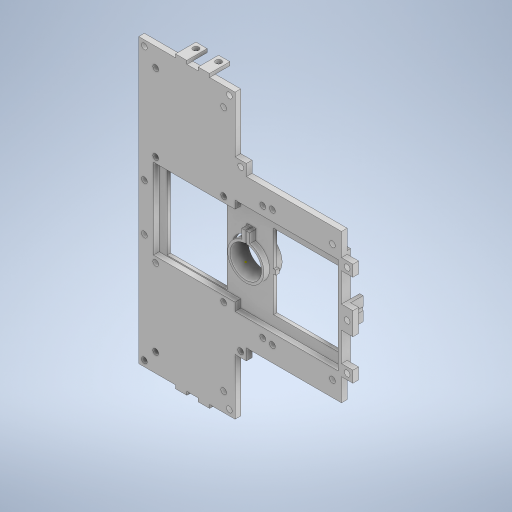
# Autodesk Inventor part: RoverMainHousing
Saved by Autodesk Inventor 2024 (Build 280153000, 153)
## iProperties
Created: 2025-11-13
Part Number: RoverMainHousing
Material: Generic
Document SubType Name: Modeling
Designer: albah
Density: 1 g/cm^3
Appearance: Default
Author: albah
Autodesk Inventor part; units mm, degrees
ref_plane "YZ Plane" through (0, 0, 0) normal (1, 0, 0) x (0, 1, 0)
ref_plane "XZ Plane" through (0, 0, 0) normal (0, 1, 0) x (-1, 0, 0)
ref_plane "XY Plane" through (0, 0, 0) normal (0, 0, 1) x (1, 0, 0)
sketch "Sketch1" plane through (0, 0, 0) normal (0, 0, 1) x (1, 0, 0)
  line L0 (-81.5, 42.5) -> (81.5, 42.5)
  line L1 (81.5, 42.5) -> (81.5, -42.5)
  line L2 (81.5, -42.5) -> (-81.5, -42.5)
  line L3 (-81.5, -42.5) -> (-81.5, 42.5)
  line L4 (-81.5, 42.5) -> (81.5, -42.5) construction
  line L5 (81.5, 42.5) -> (-81.5, -42.5) construction
  line L6 (84.5, 45.5) -> (-84.5, 45.5)
  line L7 (-84.5, 45.5) -> (-84.5, -45.5)
  line L8 (-84.5, -45.5) -> (84.5, -45.5)
  line L9 (84.5, -45.5) -> (84.5, 45.5)
  line L10 (-84.5, 45.5) -> (-84.5, 65.5)
  line L11 (-84.5, 65.5) -> (84.5, 65.5)
  line L12 (84.5, 65.5) -> (84.5, 45.5)
  line L13 (-84.5, -45.5) -> (-84.5, -65.5)
  line L14 (-84.5, -65.5) -> (84.5, -65.5)
  line L15 (84.5, -65.5) -> (84.5, -45.5)
  point P0 (0, 0)
  dimension "d0" = 163
  dimension "d1" = 85
  dimension "d4" = 3
  dimension "d167" = 20
  dimension "d168" = 20
  constraints: 32 end point, 6 perpendicular, 4 parallel, 2 midpoint, 2 point on line, 1 horizontal, 1 vertical, 3 other
  measures "d0" distance of L0.start L0.end
  measures "d1" distance of L0.end L1.end
  measures "d4" distance between parallel lines of L0 L6
  measures "d167" distance of L6.end L10.end
  measures "d168" distance of L7.end L13.end
extrude "Extrusion1" add sketch "Sketch1" along normal blind 3 contours L0 L1 L2 L3
extrude "Extrusion2" add sketch "Sketch1" along normal blind 8 contours L9 L8 L7 L6
sketch "Sketch2" plane through (0, 0, 8) normal (0, 0, 1) x (1, 0, 0)
  point P0 (0, 0)
sketch "Sketch3" plane through (0, 0, 3) normal (0, 0, 1) x (1, 0, 0)
  circle A0 centre (0, 0) radius 13.85
  circle A1 centre (0, 0) radius 16
  line L0 (0, 16) -> (0, 24)
  line L1 (0.5, 24.0267) -> (-0.5, 24.0267)
  line L2 (-0.5, 24.0267) -> (-0.5, 15.9733)
  line L3 (-0.5, 15.9733) -> (0.5, 15.9733)
  line L4 (0.5, 15.9733) -> (0.5, 24.0267)
  line L5 (0.5, 24.0267) -> (-0.5, 15.9733) construction
  line L6 (-0.5, 24.0267) -> (0.5, 15.9733) construction
  line L7 (-0.5, 24.0267) -> (-3.5, 24.0267)
  line L8 (-3.5, 24.0267) -> (-3.5, 15.6125)
  line L9 (0.5, 24.0267) -> (3.5, 24.0267)
  line L10 (3.5, 24.0267) -> (3.5, 15.6125)
  line L11 (0.5, 15.9733) -> (0.5, 13.841)
  line L12 (-0.5, 15.9733) -> (-0.5, 13.841)
  circle A2 centre (0, 0) radius 17.5
  line L13 (0, -17.5) -> (0, -16)
  line L14 (4, 15) -> (4, 25)
  line L15 (4, 25) -> (-4, 25)
  line L16 (-4, 25) -> (-4, 15)
  line L17 (-4, 15) -> (4, 15)
  line L18 (4, 15) -> (-4, 25) construction
  line L19 (4, 25) -> (-4, 15) construction
  point P0 (0, 20)
  point P1 (3.5, 17.1464)
  point P2 (4, 17.0367)
  point P3 (-4, 17.0367)
  point P4 (-3.5, 17.1464)
  point P5 (4, 15.4919)
  dimension "d15" = 35
  dimension "d7" = 27.7
  dimension "d8" = 32
  dimension "d9" = 8
  dimension "d10" = 1
  dimension "d11" = 3
  dimension "d12" = 3
  dimension "d16" = 10
  dimension "d17" = 8
  constraints: 40 end point, 6 perpendicular, 6 point on circle, 5 midpoint, 5 parallel, 3 coincident, 3 vertical, 2 centre point, 1 horizontal, 3 other
  measures "d7" diameter of A0
  measures "d8" diameter of A1
  measures "d9" distance of L0.start L0.end
  measures "d10" distance of L1.start L1.end
  measures "d11" distance of L1.end L7.end
  measures "d12" distance of L1.start L9.end
  measures "d16" distance of L14.start L14.end
  measures "d17" distance of L15.end L14.end
extrude "Extrusion3" cut sketch "Sketch3" against normal blind 8 contours A0 | A0 L12 L17 L11 | L17 L12 L3 L11 | L3 L2 A1 L4 | A1 L0 A2 L4 | L2 A2 L0 A1 | A2 L2 L1 L4 | A2 L10 L9 L1 L7 L8 L16 L15 L14
extrude "Extrusion4" cut sketch "Sketch3" against normal blind 8 contours L16 A2 L8 A1 | A1 L13 A2 L16
extrude "Extrusion5" add sketch "Sketch3" along normal blind 15 contours A0 L11 L17 L14 A1 L16 L12 | L11 L4 A1 L14 L17 | L17 L16 A1 L2 L12 | L4 A2 L10 A1 | A1 L8 A2 L2 | L4 L9 L10 A2 | A2 L8 L7 L2
extrude "Extrusion6" cut sketch "Sketch3" against normal blind 10 contours A1 L10 A2 L14
sketch "Sketch4" plane through (-3.5, 15.6125, 0) normal (-1, 0, 0) x (0, 0, 1)
  circle A0 centre (12, 4.4142) radius 2.5
  line L0 (18, 8.4142) -> (18, 0) projected
  line L1 (18, 8.4142) -> (0, 8.4142) projected
  point P0 (0, -15.6125)
  point P1 (18, 4.2071)
  dimension "d24" = 5
  dimension "d25" = 6
  dimension "d26" = 4
  constraints: 1 centre point, 1 midpoint
  measures "d24" diameter of A0
  measures "d25" horizontal distance of point (18, 4.207) A0.centre
  measures "d26" distance from line of L1 A0.centre
extrude "Extrusion7" cut sketch "Sketch4" against normal blind 10
sketch "Sketch5" plane through (0, 0, 8) normal (0, 0, 1) x (1, 0, 0)
  line L0 (84.5, -45.5) -> (84.5, 45.5) projected
  line L1 (84.5, 45.5) -> (84.5, 35.5)
  line L2 (84.5, 35.5) -> (94.5, 35.5)
  line L3 (94.5, 35.5) -> (94.5, 45.5)
  line L4 (94.5, 45.5) -> (84.5, 45.5)
  line L5 (84.5, -45.5) -> (84.5, -35.5)
  line L6 (84.5, -35.5) -> (94.5, -35.5)
  line L7 (94.5, -35.5) -> (94.5, -45.5)
  line L8 (94.5, -45.5) -> (84.5, -45.5)
  line L9 (-84.5, 45.5) -> (-84.5, -45.5) projected
  line L10 (-84.5, -45.5) -> (-84.5, -35.5)
  line L11 (-84.5, -35.5) -> (-94.5, -35.5)
  line L12 (-94.5, -35.5) -> (-94.5, -45.5)
  line L13 (-94.5, -45.5) -> (-84.5, -45.5)
  line L14 (-84.5, 45.5) -> (-84.5, 35.5)
  line L15 (-84.5, 35.5) -> (-94.5, 35.5)
  line L16 (-94.5, 35.5) -> (-94.5, 45.5)
  line L17 (-94.5, 45.5) -> (-84.5, 45.5)
  line L18 (-84.5, -45.5) -> (84.5, -45.5) projected
  line L19 (84.5, -45.5) -> (74.5, -45.5)
  line L20 (74.5, -45.5) -> (74.5, -55.5)
  line L21 (74.5, -55.5) -> (84.5, -55.5)
  line L22 (84.5, -55.5) -> (84.5, -45.5)
  line L23 (-84.5, -45.5) -> (-84.5, -55.5)
  line L24 (-84.5, -55.5) -> (-74.5, -55.5)
  line L25 (-74.5, -55.5) -> (-74.5, -45.5)
  line L26 (-74.5, -45.5) -> (-84.5, -45.5)
  line L27 (84.5, 45.5) -> (74.5, 45.5)
  line L28 (74.5, 45.5) -> (74.5, 55.5)
  line L29 (74.5, 55.5) -> (84.5, 55.5)
  line L30 (84.5, 55.5) -> (84.5, 45.5)
  line L31 (-84.5, 45.5) -> (-74.5, 45.5)
  line L32 (-74.5, 45.5) -> (-74.5, 55.5)
  line L33 (-74.5, 55.5) -> (-84.5, 55.5)
  line L34 (-84.5, 55.5) -> (-84.5, 45.5)
  line L35 (84.5, 0) -> (84.5, -10)
  line L36 (84.5, -10) -> (94.5, -10)
  line L37 (94.5, -10) -> (94.5, 0)
  line L38 (94.5, 0) -> (84.5, 0)
  line L39 (84.5, 0) -> (84.5, 10)
  line L40 (84.5, 10) -> (94.5, 10)
  line L41 (94.5, 10) -> (94.5, 0)
  line L42 (94.5, 0) -> (84.5, 0)
  line L43 (-74.5, 45.5) -> (-54.5, 45.5)
  line L44 (84.5, 45.5) -> (-84.5, 45.5) projected
  line L45 (-74.5, -45.5) -> (-54.5, -45.5)
  line L46 (-54.5, 45.5) -> (-44.5, 45.5)
  line L47 (-44.5, 45.5) -> (-44.5, 55.5)
  line L48 (-44.5, 55.5) -> (-54.5, 55.5)
  line L49 (-54.5, 55.5) -> (-54.5, 45.5)
  line L50 (-54.5, -45.5) -> (-44.5, -45.5)
  line L51 (-44.5, -45.5) -> (-44.5, -55.5)
  line L52 (-44.5, -55.5) -> (-54.5, -55.5)
  line L53 (-54.5, -55.5) -> (-54.5, -45.5)
  line L54 (74.5, 45.5) -> (54.5, 45.5)
  line L55 (74.5, -45.5) -> (54.5, -45.5)
  line L56 (54.5, -45.5) -> (44.5, -45.5)
  line L57 (44.5, -45.5) -> (44.5, -55.5)
  line L58 (44.5, -55.5) -> (54.5, -55.5)
  line L59 (54.5, -55.5) -> (54.5, -45.5)
  line L60 (54.5, 45.5) -> (44.5, 45.5)
  line L61 (44.5, 45.5) -> (44.5, 55.5)
  line L62 (44.5, 55.5) -> (54.5, 55.5)
  line L63 (54.5, 55.5) -> (54.5, 45.5)
  line L64 (0, -45.5) -> (10, -45.5)
  line L65 (0, -45.5) -> (-10, -45.5)
  line L66 (0, 45.5) -> (10, 45.5)
  line L67 (0, 45.5) -> (-10, 45.5)
  line L68 (10, -45.5) -> (20, -45.5)
  line L69 (20, -45.5) -> (20, -55.5)
  line L70 (20, -55.5) -> (10, -55.5)
  line L71 (10, -55.5) -> (10, -45.5)
  line L72 (-10, -45.5) -> (-20, -45.5)
  line L73 (-20, -45.5) -> (-20, -55.5)
  line L74 (-20, -55.5) -> (-10, -55.5)
  line L75 (-10, -55.5) -> (-10, -45.5)
  line L76 (10, 45.5) -> (20, 45.5)
  line L77 (20, 45.5) -> (20, 55.5)
  line L78 (20, 55.5) -> (10, 55.5)
  line L79 (10, 55.5) -> (10, 45.5)
  line L80 (-10, 45.5) -> (-20, 45.5)
  line L81 (-20, 45.5) -> (-20, 55.5)
  line L82 (-20, 55.5) -> (-10, 55.5)
  line L83 (-10, 55.5) -> (-10, 45.5)
  dimension "d29" = 10
  dimension "d30" = 10
  dimension "d31" = 10
  dimension "d32" = 10
  dimension "d33" = 10
  dimension "d34" = 10
  dimension "d35" = 10
  dimension "d36" = 10
  dimension "d37" = 10
  dimension "d38" = 10
  dimension "d39" = 10
  dimension "d40" = 10
  dimension "d41" = 10
  dimension "d42" = 10
  dimension "d43" = 10
  dimension "d44" = 10
  dimension "d45" = 10
  dimension "d46" = 10
  dimension "d47" = 10
  dimension "d48" = 10
  dimension "d51" = 20
  dimension "d52" = 20
  dimension "d53" = 10
  dimension "d54" = 10
  dimension "d55" = 10
  dimension "d56" = 10
  dimension "d57" = 20
  dimension "d58" = 20
  dimension "d59" = 10
  dimension "d60" = 10
  dimension "d61" = 10
  dimension "d62" = 10
  dimension "d63" = 10
  dimension "d64" = 10
  dimension "d65" = 10
  dimension "d66" = 10
  dimension "d67" = 10
  dimension "d68" = 10
  dimension "d69" = 10
  dimension "d70" = 10
  dimension "d71" = 10
  dimension "d72" = 10
  dimension "d73" = 10
  dimension "d74" = 64.5
  constraints: 160 end point, 36 parallel, 18 perpendicular, 9 point on line, 1 midpoint, 21 other
  measures "d29" distance of L0.end L1.end
  measures "d30" distance of L2.end L1.end
  measures "d31" distance of L0.start L5.end
  measures "d32" distance of L5.end L6.end
  measures "d33" distance of L9.end L10.end
  measures "d34" distance of L11.end L10.end
  measures "d35" distance of L9.start L14.end
  measures "d36" distance of L14.end L15.end
  measures "d37" distance of L0.start L19.end
  measures "d38" distance of L20.end L19.end
  measures "d39" distance of L9.end L23.end
  measures "d40" distance of L24.end L23.end
  measures "d41" distance of L0.end L27.end
  measures "d42" distance of L27.end L28.end
  measures "d43" distance of L9.start L31.end
  measures "d44" distance of L32.end L31.end
  measures "d45" distance of L35.start L35.end
  measures "d46" distance of L36.end L35.end
  measures "d47" distance of L35.start L39.end
  measures "d48" distance of L39.end L40.end
  measures "d51" distance of L31.end L43.end
  measures "d52" distance of L25.end L45.end
  measures "d53" distance of L43.end L46.end
  measures "d54" distance of L47.end L46.end
  measures "d55" distance of L45.end L50.end
  measures "d56" distance of L50.end L51.end
  measures "d57" distance of L27.end L54.end
  measures "d58" distance of L19.end L55.end
  measures "d59" distance of L55.end L56.end
  measures "d60" distance of L57.end L56.end
  measures "d61" distance of L54.end L60.end
  measures "d62" distance of L60.end L61.end
  measures "d63" distance of L64.start L64.end
  measures "d64" distance of L64.start L65.end
  measures "d65" distance of L66.start L67.end
  measures "d66" distance of L64.end L68.end
  measures "d67" distance of L68.end L69.end
  measures "d68" distance of L65.end L72.end
  measures "d69" distance of L73.end L72.end
  measures "d70" distance of L66.end L76.end
  measures "d71" distance of L77.end L76.end
  measures "d72" distance of L67.end L80.end
  measures "d73" distance of L80.end L81.end
  measures "d74" distance between parallel lines of L77 L0
extrude "Extrusion8" add sketch "Sketch5" against normal blind 5 contours L0 L6 L7 L8 | L22 L21 L20 L18 | L0 L38 L37 L36 | L59 L58 L57 L18 | L0 L40 L41 L38 | L69 L70 L71 L18 | L0 L4 L3 L2 | L27 L28 L29 L30 | L75 L74 L73 L18 | L44 L61 L62 L63 | L51 L52 L53 L18 | L44 L79 L78 L77 | L25 L24 L23 L18 | L13 L12 L11 L9 | L44 L81 L82 L83 | L15 L16 L17 L9 | L44 L49 L48 L47 | L34 L33 L32 L31
ref_plane "Work Plane1" through (0, 0, -6) normal (0, 0, -1) x (-1, 0, 0)
sketch "Sketch7" plane through (0, 0, -6) normal (0, 0, -1) x (-1, 0, 0)
  line L0 (-19.5, -35) -> (-19.5, 35)
  line L1 (-19.5, 35) -> (-79.5, 35)
  line L2 (-79.5, 35) -> (-79.5, -35)
  line L3 (-79.5, -35) -> (-19.5, -35)
  line L4 (-19.5, -35) -> (-79.5, 35) construction
  line L5 (-19.5, 35) -> (-79.5, -35) construction
  line L6 (0, 0) -> (-84.5, 0)
  line L7 (-84.5, -45.5) -> (-84.5, 45.5) projected
  line L8 (-79.5, 35) -> (-19.5, 35)
  line L9 (-19.5, 35) -> (-19.5, 33)
  line L10 (-19.5, 33) -> (-79.5, 33)
  line L11 (-79.5, 33) -> (-79.5, 35)
  line L12 (-79.5, -35) -> (-19.5, -35)
  line L13 (-19.5, -35) -> (-19.5, -33)
  line L14 (-19.5, -33) -> (-79.5, -33)
  line L15 (-79.5, -33) -> (-79.5, -35)
  line L16 (-19.5, 0) -> (-19.5, 2)
  line L17 (-19.5, 2) -> (-21.5, 2)
  line L18 (-21.5, 2) -> (-21.5, 0)
  line L19 (-21.5, 0) -> (-19.5, 0)
  line L20 (-21.5, 0) -> (-21.5, -2)
  line L21 (-16.5, 0) -> (-21.5, 0)
  line L22 (-79.5, 0) -> (-79.5, 2)
  line L23 (-79.5, 2) -> (-77.5, 2)
  line L24 (-77.5, 2) -> (-77.5, 0)
  line L25 (-77.5, 0) -> (-79.5, 0)
  line L26 (-79.5, 0) -> (-79.5, -2)
  line L27 (-79.5, -2) -> (-77.5, -2)
  line L28 (-77.5, -2) -> (-77.5, 0)
  line L29 (-77.5, 0) -> (-79.5, 0)
  line L30 (-21.5, -2) -> (-19.5, -2)
  point P0 (-49.5, 0)
  point P1 (-49.5, 0)
  point P2 (-49.5, 0)
  point P3 (-77.5, 0)
  dimension "d78" = 70
  dimension "d79" = 60
  dimension "d80" = 35
  dimension "d81" = 2
  dimension "d82" = 2
  dimension "d83" = 2
  dimension "d84" = 2
  dimension "d85" = 2
  dimension "d87" = 2
  dimension "d88" = 2
  dimension "d89" = 2
  dimension "d90" = 2
  constraints: 60 end point, 14 equal length, 8 point on line, 7 midpoint, 7 perpendicular, 1 vertical
  measures "d78" distance of L0.start L0.end
  measures "d79" distance of L1.end L0.end
  measures "d80" distance from line of L7 point (-49.5, 0)
  measures "d81" distance of L0.end L9.end
  measures "d82" distance of L13.end L0.start
  measures "d83" distance of L16.start L16.end
  measures "d84" distance of L17.end L16.end
  measures "d85" distance of L18.end L20.end
  measures "d87" distance of L22.start L22.end
  measures "d88" distance of L22.end L23.end
  measures "d89" distance of L22.start L26.end
  measures "d90" distance of L27.end L26.end
extrude "Extrusion9" cut sketch "Sketch7" against normal through all contours L14 L2 L27 L28 L6 L20 L30 L0 | L17 L18 L6 L24 L23 L2 L10 L0
extrude "Extrusion10" add sketch "Sketch7" against normal through all contours L3 L2 L14 L0 | L30 L20 L6 L0 | L6 L18 L17 L0 | L2 L6 L28 L27 | L2 L23 L24 L6 | L10 L2 L1 L0
extrude "Extrusion11" add sketch "Sketch7" along normal blind 2
sketch "Sketch8" plane through (0, 0, -6) normal (0, 0, -1) x (-1, 0, 0)
  line L0 (21.5, -37.5) -> (74.5, -37.5)
  line L1 (74.5, -37.5) -> (74.5, 37.5)
  line L2 (74.5, 37.5) -> (21.5, 37.5)
  line L3 (21.5, 37.5) -> (21.5, -37.5)
  line L4 (21.5, -37.5) -> (74.5, 37.5) construction
  line L5 (74.5, -37.5) -> (21.5, 37.5) construction
  line L6 (0, 0) -> (84.5, 0)
  line L7 (84.5, 35.5) -> (84.5, -35.5) projected
  line L8 (-84.5, 45.5) -> (84.5, 45.5) projected
  line L9 (21.5, 37.5) -> (74.5, 37.5)
  line L10 (74.5, 37.5) -> (74.5, 34.5)
  line L11 (74.5, 34.5) -> (21.5, 34.5)
  line L12 (21.5, 34.5) -> (21.5, 37.5)
  line L13 (21.5, -37.5) -> (74.5, -37.5)
  line L14 (74.5, -37.5) -> (74.5, -34.5)
  line L15 (74.5, -34.5) -> (21.5, -34.5)
  line L16 (21.5, -34.5) -> (21.5, -37.5)
  line L17 (77.5, -37.5) -> (77.5, 37.5)
  line L18 (74.5, 37.5) -> (77.5, 37.5)
  line L19 (74.5, -37.5) -> (77.5, -37.5)
  point P0 (48, 0)
  point P1 (48, 0)
  point P2 (77.5, 0)
  point P3 (74.5, 0)
  dimension "d97" = 10
  dimension "d98" = 8
  dimension "d99" = 53
  dimension "d100" = 3
  dimension "d101" = 3
  dimension "d102" = 3
  constraints: 36 end point, 9 equal length, 4 midpoint, 4 perpendicular, 2 horizontal, 1 point on line
  measures "d97" distance between parallel lines of L7 L1
  measures "d98" distance between parallel lines of L8 L2
  measures "d99" distance of L1.end L2.end
  measures "d100" distance of L1.end L10.end
  measures "d101" distance of L14.end L0.end
  measures "d102" distance between parallel lines of L1 L17
extrude "Extrusion12" cut sketch "Sketch8" against normal through all contours L3 L6 L1 L15 | L3 L11 L1 L6
extrude "Extrusion13" add sketch "Sketch8" against normal through all contours L3 L15 L1 L0 | L3 L2 L1 L11
extrude "Extrusion15" add sketch "Sketch8" against normal blind 2 contours L3 L6 L1 L15 | L3 L11 L1 L6
extrude "Extrusion17" add sketch "Sketch1" along normal up to surface (8 mm away) contours L6 L10 L11 L12 | L15 L14 L13 L8
extrude "Extrusion18" cut sketch "Sketch1" along normal blind 3 contours L6 L10 L11 L12 | L15 L14 L13 L8
sketch "Sketch9" plane through (0, 0, 8) normal (0, 0, 1) x (1, 0, 0)
  circle A0 centre (79.5, -50.5) radius 2.5
  circle A1 centre (49.5, -50.5) radius 2.5
  circle A2 centre (15, -50.5) radius 2.5
  circle A3 centre (-15, -50.5) radius 2.5
  circle A4 centre (-49.5, -50.5) radius 2.5
  circle A5 centre (-79.5, -50.5) radius 2.5
  circle A6 centre (-89.5, -40.5) radius 2.5
  circle A7 centre (-89.5, 40.5) radius 2.5
  circle A8 centre (-79.5, 50.5) radius 2.5
  circle A9 centre (-49.5, 50.5) radius 2.5
  circle A10 centre (-15, 50.5) radius 2.5
  circle A11 centre (15, 50.5) radius 2.5
  circle A12 centre (49.5, 50.5) radius 2.5
  circle A13 centre (79.5, 50.5) radius 2.5
  circle A14 centre (89.5, 40.5) radius 2.5
  circle A15 centre (89.5, 5) radius 2.5
  circle A16 centre (89.5, -5) radius 2.5
  circle A17 centre (89.5, -40.5) radius 2.5
  line L0 (84.5, -55.5) -> (84.5, -45.5) projected
  line L1 (74.5, -55.5) -> (84.5, -55.5) projected
  line L2 (44.5, -55.5) -> (54.5, -55.5) projected
  line L3 (54.5, -55.5) -> (54.5, -45.5) projected
  line L4 (10, -55.5) -> (20, -55.5) projected
  line L5 (20, -55.5) -> (20, -45.5) projected
  line L6 (-20, -55.5) -> (-10, -55.5) projected
  line L7 (-10, -55.5) -> (-10, -45.5) projected
  line L8 (-54.5, -55.5) -> (-44.5, -55.5) projected
  line L9 (-44.5, -55.5) -> (-44.5, -45.5) projected
  line L10 (-84.5, -55.5) -> (-74.5, -55.5) projected
  line L11 (-74.5, -55.5) -> (-74.5, -45.5) projected
  line L12 (-94.5, -45.5) -> (-84.5, -45.5) projected
  line L13 (-94.5, -35.5) -> (-94.5, -45.5) projected
  line L14 (-84.5, 45.5) -> (-94.5, 45.5) projected
  line L15 (-94.5, 45.5) -> (-94.5, 35.5) projected
  line L16 (-74.5, 45.5) -> (-74.5, 55.5) projected
  line L17 (-74.5, 55.5) -> (-84.5, 55.5) projected
  line L18 (-44.5, 55.5) -> (-54.5, 55.5) projected
  line L19 (-44.5, 45.5) -> (-44.5, 55.5) projected
  line L20 (-10, 55.5) -> (-20, 55.5) projected
  line L21 (-10, 45.5) -> (-10, 55.5) projected
  line L22 (20, 55.5) -> (10, 55.5) projected
  line L23 (20, 45.5) -> (20, 55.5) projected
  line L24 (54.5, 55.5) -> (44.5, 55.5) projected
  line L25 (54.5, 45.5) -> (54.5, 55.5) projected
  line L26 (84.5, 55.5) -> (74.5, 55.5) projected
  line L27 (84.5, 45.5) -> (84.5, 55.5) projected
  line L28 (94.5, 45.5) -> (84.5, 45.5) projected
  line L29 (94.5, 35.5) -> (94.5, 45.5) projected
  line L30 (94.5, 10) -> (84.5, 10) projected
  line L31 (94.5, -10) -> (94.5, 10) projected
  line L32 (84.5, -10) -> (94.5, -10) projected
  line L33 (94.5, -45.5) -> (94.5, -35.5) projected
  line L34 (84.5, -45.5) -> (94.5, -45.5) projected
  point P0 (0, 0)
  point P1 (79.5, -55.5)
  point P2 (49.5, -55.5)
  point P3 (54.5, -50.5)
  point P4 (15, -55.5)
  point P5 (20, -50.5)
  point P6 (-15, -55.5)
  point P7 (-10, -50.5)
  point P8 (-49.5, -55.5)
  point P9 (-44.5, -50.5)
  point P10 (-79.5, -55.5)
  point P11 (-89.5, -45.5)
  point P12 (-94.5, -40.5)
  point P13 (-89.5, 45.5)
  point P14 (-94.5, 40.5)
  point P15 (-74.5, 50.5)
  point P16 (-79.5, 55.5)
  point P17 (-49.5, 55.5)
  point P18 (-44.5, 50.5)
  point P19 (-15, 55.5)
  point P20 (-10, 50.5)
  point P21 (15, 55.5)
  point P22 (20, 50.5)
  point P23 (49.5, 55.5)
  point P24 (54.5, 50.5)
  point P25 (79.5, 55.5)
  point P26 (84.5, 50.5)
  point P27 (89.5, 45.5)
  point P28 (94.5, 40.5)
  point P29 (89.5, 10)
  point P30 (89.5, -10)
  point P31 (94.5, -40.5)
  dimension "d111" = 5
  dimension "d112" = 5
  dimension "d113" = 5
  dimension "d114" = 5
  dimension "d115" = 5
  dimension "d116" = 5
  dimension "d117" = 5
  dimension "d118" = 5
  dimension "d119" = 5
  dimension "d120" = 5
  dimension "d121" = 5
  dimension "d122" = 5
  dimension "d123" = 5
  dimension "d124" = 5
  dimension "d125" = 5
  dimension "d126" = 5
  dimension "d127" = 5
  dimension "d128" = 5
  dimension "d129" = 5
  dimension "d130" = 5
  dimension "d131" = 5
  dimension "d132" = 5
  dimension "d133" = 5
  dimension "d134" = 5
  dimension "d135" = 5
  dimension "d136" = 5
  dimension "d137" = 5
  dimension "d138" = 5
  dimension "d139" = 5
  dimension "d140" = 5
  dimension "d141" = 5
  dimension "d142" = 5
  dimension "d143" = 5
  dimension "d144" = 5
  dimension "d145" = 5
  dimension "d146" = 5
  dimension "d147" = 5
  dimension "d148" = 5
  dimension "d149" = 5
  dimension "d150" = 5
  dimension "d151" = 5
  dimension "d152" = 5
  dimension "d153" = 5
  dimension "d154" = 5
  dimension "d155" = 5
  dimension "d156" = 5
  dimension "d157" = 5
  dimension "d158" = 5
  dimension "d159" = 5
  dimension "d160" = 5
  dimension "d161" = 5
  dimension "d162" = 5
  dimension "d163" = 5
  dimension "d164" = 5
  constraints: 31 midpoint, 18 centre point
  measures "d111" diameter of A0
  measures "d112" diameter of A1
  measures "d113" diameter of A2
  measures "d114" diameter of A3
  measures "d115" diameter of A4
  measures "d116" diameter of A5
  measures "d117" diameter of A6
  measures "d118" diameter of A7
  measures "d119" diameter of A8
  measures "d120" diameter of A9
  measures "d121" diameter of A10
  measures "d122" diameter of A11
  measures "d123" diameter of A12
  measures "d124" diameter of A13
  measures "d125" diameter of A14
  measures "d126" diameter of A15
  measures "d127" diameter of A16
  measures "d128" diameter of A17
  measures "d129" distance from line of L0 A0.centre
  measures "d130" distance of point (79.5, -55.5) A0.centre
  measures "d131" distance of point (49.5, -55.5) A1.centre
  measures "d132" distance of point (54.5, -50.5) A1.centre
  measures "d133" distance of point (15, -55.5) A2.centre
  measures "d134" distance of point (20, -50.5) A2.centre
  measures "d135" distance of point (-15, -55.5) A3.centre
  measures "d136" distance of point (-10, -50.5) A3.centre
  measures "d137" distance of point (-49.5, -55.5) A4.centre
  measures "d138" distance of point (-44.5, -50.5) A4.centre
  measures "d139" distance of point (-79.5, -55.5) A5.centre
  measures "d140" distance from line of L11 A5.centre
  measures "d141" distance of point (-89.5, -45.5) A6.centre
  measures "d142" distance of point (-94.5, -40.5) A6.centre
  measures "d143" distance of point (-89.5, 45.5) A7.centre
  measures "d144" distance of point (-94.5, 40.5) A7.centre
  measures "d145" distance of point (-74.5, 50.5) A8.centre
  measures "d146" distance of point (-79.5, 55.5) A8.centre
  measures "d147" distance of point (-49.5, 55.5) A9.centre
  measures "d148" distance of point (-44.5, 50.5) A9.centre
  measures "d149" distance of point (-15, 55.5) A10.centre
  measures "d150" distance of point (-10, 50.5) A10.centre
  measures "d151" distance of point (15, 55.5) A11.centre
  measures "d152" distance of point (20, 50.5) A11.centre
  measures "d153" distance of A12.centre point (49.5, 55.5)
  measures "d154" distance of point (54.5, 50.5) A12.centre
  measures "d155" distance of A13.centre point (79.5, 55.5)
  measures "d156" distance of point (84.5, 50.5) A13.centre
  measures "d157" distance of A14.centre point (89.5, 45.5)
  measures "d158" distance of A14.centre point (94.5, 40.5)
  measures "d159" distance of point (89.5, 10) A15.centre
  measures "d160" distance from line of L31 A15.centre
  measures "d161" distance of point (89.5, -10) A16.centre
  measures "d162" distance from line of L31 A16.centre
  measures "d163" distance of point (94.5, -40.5) A17.centre
  measures "d164" distance from line of L34 A17.centre
extrude "Extrusion16" cut sketch "Sketch9" against normal blind 10 contours A2 | A3 | A4 | A5 | A6 | A7 | A8 | A9 | A10 | A11
move faces "Move1" translate (0, 0, 8) faces at (39.5, -11.6667, -8)
move faces "Move2" translate (0, 0, 6) faces at (-56.8333, 11.5, -6) (-39.1667, 35.5, -6) (-56.8333, -35.5, -6)
sketch "Sketch10" plane through (-84.5, -35.5, 8) normal (-1, 0, 0) x (0, 0, 1)
  line L0 (-16, 45.5) -> (-16, 25.5)
  line L1 (-16, 25.5) -> (0, 25.5)
  line L2 (0, 25.5) -> (0, 45.5)
  line L3 (0, 45.5) -> (-16, 45.5)
  line L4 (-16, 45.5) -> (0, 25.5) construction
  line L5 (-16, 25.5) -> (0, 45.5) construction
  point P0 (-8, 35.5)
  dimension "d179" = 20
  dimension "d180" = 38.66
  constraints: 12 end point, 2 midpoint, 2 parallel, 1 horizontal, 1 perpendicular
  measures "d179" distance of L0.start L0.end
  measures "d180" angle of L4 L2
extrude "Extrusion19" add sketch "Sketch10" along normal blind 3
sketch "Sketch11" plane through (-84.5, 45.5, 3) normal (0, 1, 0) x (1, 0, 0)
  line L0 (84.5, 3) -> (68.5, 3) projected
  line L1 (84.5, 3) -> (74.5, 3)
  line L2 (74.5, 3) -> (74.5, 11)
  line L3 (74.5, 11) -> (84.5, 11)
  line L4 (84.5, 11) -> (84.5, 3)
  line L5 (84.5, 3) -> (94.5, 3)
  line L6 (94.5, 3) -> (94.5, 11)
  line L7 (94.5, 11) -> (84.5, 11)
  line L8 (84.5, 11) -> (84.5, 3)
  line L9 (94.5, 3) -> (74.5, 3)
  line L10 (74.5, 3) -> (74.5, 0)
  line L11 (74.5, 0) -> (94.5, 0)
  line L12 (94.5, 0) -> (94.5, 3)
  point P0 (81, 3)
  dimension "d183" = 10
  dimension "d184" = 8
  dimension "d185" = 10
  dimension "d186" = 8
  constraints: 24 end point, 6 parallel, 3 perpendicular, 2 point on line, 1 collinear
  measures "d183" distance of L0.start L1.end
  measures "d184" distance of L1.end L2.end
  measures "d185" distance of L0.start L5.end
  measures "d186" distance of L6.end L5.end
extrude "Extrusion20" add sketch "Sketch11" along normal blind 3
sketch "Sketch12" plane through (-84.5, -45.5, 3) normal (0, -1, 0) x (1, 0, 0)
  line L0 (94.5, -11) -> (74.5, -11) projected
  line L1 (74.5, -11) -> (94.5, -11)
  line L2 (94.5, -11) -> (94.5, 0)
  line L3 (94.5, 0) -> (74.5, 0)
  line L4 (74.5, 0) -> (74.5, -11)
  point P0 (84.5, -3)
  constraints: 8 end point, 3 equal length, 1 perpendicular
extrude "Extrusion21" add sketch "Sketch12" along normal blind 3
sketch "Sketch13" plane through (84.5, 10, 8) normal (1, 0, 0) x (0, 0, -1)
  line L0 (16, 0) -> (16, -20) projected
  line L1 (16, -20) -> (16, 0)
  line L2 (16, 0) -> (0, 0)
  line L3 (0, 0) -> (0, -20)
  line L4 (0, -20) -> (16, -20)
  point P0 (8, -10)
  constraints: 8 end point, 3 equal length, 1 perpendicular
extrude "Extrusion22" add sketch "Sketch13" along normal blind 3
move faces "Move3" translate (0, 0, -3) faces at (-16.3996, 61.3273, 3) (-4.8996, -61.3273, 3)
sketch "Sketch14" plane through (0, 0, 8) normal (0, 0, 1) x (1, 0, 0)
  line L0 (23.5, -51.75) -> (23.5, 51.75)
  line L1 (23.5, 51.75) -> (76.5, 51.75)
  line L2 (76.5, 51.75) -> (76.5, -51.75)
  line L3 (76.5, -51.75) -> (23.5, -51.75)
  line L4 (23.5, -51.75) -> (76.5, 51.75) construction
  line L5 (23.5, 51.75) -> (76.5, -51.75) construction
  circle A0 centre (23.5, 51.75) radius 2.5
  circle A1 centre (76.5, 51.75) radius 2.5
  circle A2 centre (76.5, -51.75) radius 2.5
  circle A3 centre (23.5, -51.75) radius 2.5
  point P0 (0, 0)
  point P1 (50, 0)
  point P2 (50, 0)
  dimension "d196" = 103.5
  dimension "d197" = 53
  dimension "d198" = 50
  dimension "d199" = 76.5
  dimension "d200" = 5
  dimension "d201" = 5
  dimension "d202" = 5
  dimension "d203" = 5
  constraints: 12 end point, 4 centre point, 4 coincident, 3 midpoint, 2 parallel, 1 perpendicular, 1 vertical
  measures "d196" distance of L0.start L0.end
  measures "d197" distance of L0.end L1.end
  measures "d198" distance of point (0, 0) point (50, 0)
  measures "d199" distance from line of point (0, 0) L2
  measures "d200" diameter of A0
  measures "d201" diameter of A1
  measures "d202" diameter of A2
  measures "d203" diameter of A3
extrude "Extrusion23" cut sketch "Sketch14" against normal through all contours L3 A3 L0 | L0 A3 L3 | A0 L1 L0 | L0 L1 A0 | A2 L2 L3 | L3 L2 A2 | A1 L2 L1 | L1 L2 A1
sketch "Sketch15" plane through (0, 0, 8) normal (0, 0, 1) x (1, 0, 0)
  line L0 (-16, 36) -> (-16, 113)
  line L1 (-16, 113) -> (-83, 113)
  line L2 (-83, 113) -> (-83, 36)
  line L3 (-83, 36) -> (-16, 36)
  line L4 (-16, 36) -> (-83, 113) construction
  line L5 (-16, 113) -> (-83, 36) construction
  line L6 (84.5, -65.5) -> (-84.5, -65.5) projected
  line L7 (-84.5, 65.5) -> (-84.5, 45.5) projected
  line L8 (-84.5, 65.5) -> (-84.5, 113)
  line L9 (-84.5, 113) -> (-83, 113)
  line L10 (-84.5, 65.5) -> (-83, 65.5)
  line L11 (-94.5, 45.5) -> (-94.5, 35.5) projected
  line L12 (-94.5, 35.5) -> (-94.5, 113)
  line L13 (-94.5, 113) -> (-9.5, 113)
  line L14 (-9.5, 113) -> (-9.5, 35.5)
  line L15 (-9.5, 35.5) -> (-94.5, 35.5)
  line L16 (-19.5, 40.5) -> (-19.5, 108.5)
  line L17 (-19.5, 108.5) -> (-79.5, 108.5)
  line L18 (-79.5, 108.5) -> (-79.5, 40.5)
  line L19 (-79.5, 40.5) -> (-19.5, 40.5)
  line L20 (-19.5, 40.5) -> (-79.5, 108.5) construction
  line L21 (-19.5, 108.5) -> (-79.5, 40.5) construction
  circle A0 centre (-79.5, 108.5) radius 2.5
  circle A1 centre (-79.5, 40.5) radius 2.5
  circle A2 centre (-19.5, 40.5) radius 2.5
  circle A3 centre (-19.5, 108.5) radius 2.5
  line L22 (-94.5, 113) -> (-9.5, 113)
  line L23 (-9.5, 113) -> (-9.5, 125)
  line L24 (-9.5, 125) -> (-94.5, 125)
  line L25 (-94.5, 125) -> (-94.5, 113)
  point P0 (0, 0)
  point P1 (-49.5, 74.5)
  point P2 (-49.5, 74.5)
  dimension "d206" = 77
  dimension "d207" = 67
  dimension "d208" = 140
  dimension "d209" = 85
  dimension "d210" = 68
  dimension "d211" = 60
  dimension "d212" = 5
  dimension "d213" = 5
  dimension "d214" = 5
  dimension "d215" = 5
  dimension "d216" = 68.5
  dimension "d217" = 178.5
  dimension "d222" = 12
  constraints: 46 end point, 8 parallel, 6 perpendicular, 5 midpoint, 4 centre point, 4 coincident, 3 vertical, 2 collinear, 1 point on line
  measures "d206" distance of L0.start L0.end
  measures "d207" distance of L1.end L0.end
  measures "d208" distance from line of L6 point (-49.5, 74.5)
  measures "d209" distance of L12.end L13.end
  measures "d210" distance of L16.start L16.end
  measures "d211" distance of L17.end L16.end
  measures "d212" diameter of A0
  measures "d213" diameter of A1
  measures "d214" diameter of A2
  measures "d215" diameter of A3
  measures "d216" distance between parallel lines of L7 L0
  measures "d217" distance between parallel lines of L13 L6
  measures "d222" distance of L23.end L13.end
extrude "Extrusion24" add sketch "Sketch15" against normal up to surface (8 mm away) contours L3 L2 L1 L0 | L0 L13 L14 L15 L11 L12 L8 L10 L2 L3 | L1 L9 L13 L25 L24 L23 | L2 L10 L8 L9 | L19 A2 L16 | L16 A2 L19 | A2 L19 A1 L18 A0 L17 A3 L16 | A3 L17 L16 | L16 L17 A3 | A1 L18 L19 | L19 L18 A1 | A0 L18 L17 | L17 L18 A0
extrude "Extrusion25" cut sketch "Sketch15" against normal through all contours L19 A2 L16 | L16 A2 L19 | A3 L17 L16 | L16 L17 A3 | A1 L18 L19 | L19 L18 A1 | A0 L18 L17 | L17 L18 A0
mirror "Mirror1" about plane through (0, 0, 0) normal (0, 1, 0) of "Extrusion24", "Extrusion25"
sketch "Sketch16" plane through (-94.5, -125, 8) normal (0, -1, 0) x (1, 0, 0)
  line L0 (0, -8) -> (85, -8) projected
  line L1 (42.5, -8) -> (52.5, -8)
  line L2 (52.5, -8) -> (62.5, -8)
  line L3 (62.5, -8) -> (62.5, -18)
  line L4 (62.5, -18) -> (52.5, -18)
  line L5 (52.5, -18) -> (52.5, -8)
  line L6 (52.5, -8) -> (62.5, -8)
  line L7 (62.5, -8) -> (62.5, 0)
  line L8 (62.5, 0) -> (52.5, 0)
  line L9 (52.5, 0) -> (52.5, -8)
  line L10 (85, 0) -> (0, 0) projected
  line L11 (42.5, 0) -> (42.5, -18)
  line L12 (42.5, -18) -> (32.5, -18)
  line L13 (32.5, -18) -> (32.5, 0)
  line L14 (32.5, 0) -> (42.5, 0)
  circle A0 centre (37.5, -13) radius 2.5
  circle A1 centre (57.5, -13) radius 2.5
  point P0 (94.5, -8)
  point P1 (32.5, 0)
  dimension "d223" = 10
  dimension "d224" = 10
  dimension "d225" = 10
  dimension "d226" = 10
  dimension "d227" = 0
  dimension "d228" = 5
  dimension "d229" = 5
  dimension "d230" = 5
  dimension "d231" = 5
  dimension "d232" = 13
  dimension "d233" = 5
  constraints: 26 end point, 6 parallel, 4 perpendicular, 3 point on line, 2 centre point, 2 midpoint, 1 collinear
  measures "d223" distance of L1.start L1.end
  measures "d224" distance of L1.end L2.end
  measures "d225" distance of L2.end L3.end
  measures "d226" distance of L11.end L12.end
  measures "d227" distance between parallel lines of L8 L10
  measures "d228" diameter of A0
  measures "d229" diameter of A1
  measures "d230" distance from line of L12 A0.centre
  measures "d231" distance from line of L13 A0.centre
  measures "d232" distance from line of A1.centre L10
  measures "d233" distance from line of A1.centre L7
extrude "Extrusion26" add sketch "Sketch16" along normal blind 3 contours L11 L12 L13 L0 | L0 L13 L10 L11 | L9 L8 L7 L0 | L0 L3 L4 L5
mirror "Mirror2" about plane through (0, 0, 0) normal (0, 1, 0) of "Extrusion26"
sketch "Sketch17" plane through (0, 0, 8) normal (0, 0, 1) x (1, 0, 0)
  line L0 (-84.5, 35.5) -> (-94.5, 35.5) projected
  line L1 (-89.5, 35.5) -> (-89.5, 0)
  line L2 (-89.5, 0) -> (0, 0)
  line L3 (-94.5, 125) -> (-62, 125) projected
  circle A0 centre (-89.5, 120) radius 2.5
  circle A1 centre (-14.5, 120) radius 2.5
  line L4 (-9.5, 125) -> (-32, 125) projected
  line L5 (-9.5, 65.5) -> (-9.5, 125) projected
  line L6 (-94.5, 125) -> (-94.5, 35.5) projected
  line L7 (-84.5, 35.5) -> (-84.5, 10) projected
  line L8 (-94.5, 35.5) -> (-84.5, 35.5)
  line L9 (-84.5, 35.5) -> (-84.5, -41.5)
  line L10 (-84.5, -41.5) -> (-94.5, -41.5)
  line L11 (-94.5, -41.5) -> (-94.5, 35.5)
  circle A2 centre (-89.5, 17.75) radius 2.5
  circle A3 centre (-89.5, -23.75) radius 2.5
  line L12 (-9.5, 65.5) -> (84.5, 65.5) projected
  line L13 (-9.5, 65.5) -> (0.5, 65.5)
  line L14 (0.5, 65.5) -> (0.5, 75.5)
  line L15 (0.5, 75.5) -> (-9.5, 75.5)
  line L16 (-9.5, 75.5) -> (-9.5, 65.5)
  circle A4 centre (-4.5, 70.5) radius 2.5
  circle A5 centre (89.5, 40.5) radius 2.5
  line L17 (94.5, 45.5) -> (84.5, 45.5) projected
  line L18 (94.5, 35.5) -> (94.5, 45.5) projected
  circle A6 centre (89.5, 0) radius 2.5
  line L19 (94.5, -10) -> (94.5, 10) projected
  line L20 (94.5, 10) -> (84.5, 10) projected
  point P0 (-89.5, -41.5)
  point P1 (89.5, 45.5)
  dimension "d238" = 5
  dimension "d240" = 5
  dimension "d241" = 5
  dimension "d242" = 5
  dimension "d243" = 5
  dimension "d244" = 5
  dimension "d247" = 5
  dimension "d248" = 166.5
  dimension "d249" = 5
  dimension "d250" = 17.75
  dimension "d251" = 5
  dimension "d252" = 10
  dimension "d253" = 10
  dimension "d254" = 5
  dimension "d255" = 5
  dimension "d256" = 80
  dimension "d257" = 5
  dimension "d258" = 5
  dimension "d259" = 5
  dimension "d264" = 5
  dimension "d265" = 5
  dimension "d266" = 10
  constraints: 20 end point, 7 centre point, 4 midpoint, 4 parallel, 3 perpendicular, 1 horizontal, 1 point on line, 1 vertical
  measures "d238" diameter of A0
  measures "d240" diameter of A1
  measures "d241" distance from line of L4 A1.centre
  measures "d242" distance from line of L5 A1.centre
  measures "d243" distance from line of L3 A0.centre
  measures "d244" distance from line of L6 A0.centre
  measures "d247" diameter of A2
  measures "d248" distance between parallel lines of L4 L10
  measures "d249" diameter of A3
  measures "d250" distance of point (-89.5, -41.5) A3.centre
  measures "d251" distance from line of L11 A3.centre
  measures "d252" distance of L5.start L13.end
  measures "d253" distance of L14.end L13.end
  measures "d254" diameter of A4
  measures "d255" distance from line of A4.centre L12
  measures "d256" distance from line of A4.centre L7
  measures "d257" diameter of A5
  measures "d258" distance of point (89.5, 45.5) A5.centre
  measures "d259" distance from line of L18 A5.centre
  measures "d264" diameter of A6
  measures "d265" distance from line of L19 A6.centre
  measures "d266" distance from line of L20 A6.centre
extrude "Extrusion27" add sketch "Sketch17" against normal blind 5 contours L7 L9 L2 L1 A2 L0 | L1 A2 L2 L9 L10 L11 L0 | L5 L15 L14 L12
extrude "Extrusion28" cut sketch "Sketch17" against normal through all contours A0 | A1 | A4 | A5 | A6
mirror "Mirror3" about plane through (0, 0, 0) normal (0, 1, 0) of "Extrusion28", "Extrusion27"
move faces "Move4" translate (0, 0, -10) faces at (1.5, 17.8267, 18)
extrude "Extrusion29" add sketch "Sketch3" against normal blind 5 contours A0 L11 L17 L14 A1 L16 L12 | L11 L4 A1 L14 L17 | L17 L16 A1 L2 L12 | L4 A2 L10 A1 | A1 L8 A2 L2 | L4 L9 L10 A2 | A2 L8 L7 L2
move faces "Move5" translate (0, 0, -6) faces at (2.5, 18.5375, -2)
sketch "Sketch18" plane through (-3.5, 15.6125, 8) normal (-1, 0, 0) x (0, 0, 1)
  circle A0 centre (-12, 4.4142) radius 2.5
  line L0 (0, 8.4142) -> (-16, 8.4142) projected
  line L1 (-16, 0) -> (-16, 8.4142) projected
  point P0 (-8, -15.6125)
  dimension "d275" = 5
  dimension "d276" = 4
  dimension "d277" = 4
  constraints: 1 centre point
  measures "d275" diameter of A0
  measures "d276" distance from line of L0 A0.centre
  measures "d277" distance from line of L1 A0.centre
extrude "Extrusion30" cut sketch "Sketch18" against normal blind 10
extrude "Extrusion31" cut sketch "Sketch17" against normal blind 5 contours A2 L1 | L1 A2 | A3
sketch "Sketch19" plane through (84.5, 10, 0) normal (0, 0, -1) x (-1, 0, 0)
  line L0 (0, 35.5) -> (169, 35.5)
  line L1 (169, 35.5) -> (169, -55.5)
  line L2 (169, -55.5) -> (0, -55.5)
  line L3 (0, -55.5) -> (0, 35.5)
  line L4 (0, 35.5) -> (169, -55.5) construction
  line L5 (169, 35.5) -> (0, -55.5) construction
  line L6 (172, -58.5) -> (172, 38.5)
  line L7 (172, 38.5) -> (-3, 38.5)
  line L8 (-3, 38.5) -> (-3, -58.5)
  line L9 (-3, -58.5) -> (172, -58.5)
  line L10 (223.8377, 138.8608) -> (-54.8377, 138.8608)
  line L11 (-54.8377, 138.8608) -> (-54.8377, -158.8608)
  line L12 (-54.8377, -158.8608) -> (223.8377, -158.8608)
  line L13 (223.8377, -158.8608) -> (223.8377, 138.8608)
  line L14 (223.8377, 138.8608) -> (-54.8377, -158.8608) construction
  line L15 (-54.8377, 138.8608) -> (223.8377, -158.8608) construction
  line L16 (146.5, 118) -> (136.5, 118) projected
  line L17 (146.5, 115) -> (136.5, 115) projected
  line L18 (146.5, 118) -> (146.5, 115)
  line L19 (146.5, 115) -> (136.5, 115)
  line L20 (136.5, 115) -> (136.5, 118)
  line L21 (136.5, 118) -> (146.5, 118)
  line L22 (126.5, 115) -> (126.5, 118) projected
  line L23 (126.5, 118) -> (126.5, 115)
  line L24 (126.5, 115) -> (116.5, 115)
  line L25 (116.5, 115) -> (116.5, 118)
  line L26 (116.5, 118) -> (126.5, 118)
  line L27 (136.5, -138) -> (146.5, -138) projected
  line L28 (146.5, -135) -> (136.5, -135) projected
  line L29 (146.5, -138) -> (146.5, -135)
  line L30 (146.5, -135) -> (136.5, -135)
  line L31 (136.5, -135) -> (136.5, -138)
  line L32 (136.5, -138) -> (146.5, -138)
  line L33 (126.5, -138) -> (126.5, -135)
  line L34 (126.5, -135) -> (116.5, -135)
  line L35 (116.5, -135) -> (116.5, -138)
  line L36 (116.5, -138) -> (126.5, -138)
  point P0 (84.5, -10)
  dimension "d282" = 3
  constraints: 64 end point, 15 equal length, 10 perpendicular, 4 midpoint, 4 point on line, 3 other
  measures "d282" distance between parallel lines of L1 L6
extrude "Extrusion32" cut sketch "Sketch19" against normal blind 3 contours L13 L12 L11 L10
sketch "Sketch20" plane through (-84.5, -35.5, 0) normal (0, 0, -1) x (-1, 0, 0)
  circle A0 centre (-161, 87.25) radius 2.5 projected
  circle A1 centre (-161, 87.25) radius 5.5
  arc A2 (-98, 84) -> (-101, 84) centre (-99.5, 86) ccw projected
  circle A3 centre (-99.5, 86) radius 5
  circle A4 centre (-99.5, -15) radius 2.5 projected
  circle A5 centre (-99.5, -15) radius 5
  circle A6 centre (-161, -16.25) radius 2.5 projected
  circle A7 centre (-161, -16.25) radius 5.5
  point P0 (-84.5, 35.5)
  dimension "d285" = 11
  dimension "d286" = 10
  dimension "d287" = 10
  dimension "d288" = 11
  constraints: 4 centre point, 4 coincident
  measures "d285" diameter of A1
  measures "d286" diameter of A3
  measures "d287" diameter of A5
  measures "d288" diameter of A7
extrude "Extrusion33" cut sketch "Sketch20" against normal blind 3
fillet "Fillet1" radius 2 4 edges at (-38.5413, 48.5, 3) (45.8228, 48.5, 3) (45.8228, -48.5, 3) (-38.5413, -48.5, 3)
body "Solid1"
